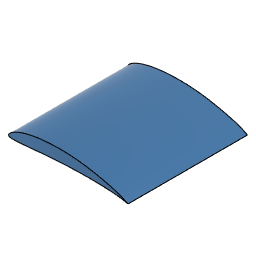
AH79100c Airfoil v1 (Autodesk Fusion 360 design; units mm, degrees)
Autodesk Fusion 360 part; units mm, degrees
sketch "AH_79-100_C_AIRFOIL_1.0" plane through (0, 0, 0) normal (0, 1, 0) x (1, 0, 0)
  spline S0 degree 5 poles (100, 0) (100.0003, -0.0014) (99.9852, -0.0078) (99.9152, -0.0286) (99.7881, -0.0733) (99.6465, -0.1452) (99.4909, -0.2271) (99.3022, -0.3153) (99.0882, -0.4084) (98.8641, -0.5062) (98.6365, -0.6097) (98.4042, -0.7199) (98.1633, -0.8374) (97.9114, -0.9618) (97.649, -1.0915) (97.3779, -1.2244) (97.1, -1.3589) (96.8164, -1.4941) (96.527, -1.6299) (96.2315, -1.7664) (95.9296, -1.9037) (95.6211, -2.0415) (95.3062, -2.1791) (94.9853, -2.3159) (94.6587, -2.4513) (94.3268, -2.5849) (93.9898, -2.7169) (93.6478, -2.8474) (93.3009, -2.9767) (92.9492, -3.1051) (92.5929, -3.2325) (92.2321, -3.359) (91.867, -3.4845) (91.4977, -3.6088) (91.1244, -3.7319) (90.7472, -3.854) (90.3662, -3.9753) (89.9815, -4.096) (89.5933, -4.2164) (89.2015, -4.3365) (88.8063, -4.4563) (88.4078, -4.5759) (88.0061, -4.6951) (87.6012, -4.8137) (87.1932, -4.9318) (86.7822, -5.0492) (86.3683, -5.166) (85.9515, -5.2822) (85.532, -5.3979) (85.1098, -5.5131) (84.6848, -5.6277) (84.2573, -5.7418) (83.8272, -5.8553) (83.3947, -5.9681) (82.9596, -6.0802) (82.5222, -6.1916) (82.0824, -6.3022) (81.6404, -6.4121) (81.1961, -6.5214) (80.7496, -6.6301) (80.3011, -6.7381) (79.8505, -6.8456) (79.3978, -6.9525) (78.9432, -7.0587) (78.4866, -7.1642) (78.0281, -7.269) (77.5676, -7.3728) (77.1054, -7.4759) (76.6413, -7.578) (76.1754, -7.6792) (75.7078, -7.7796) (75.2385, -7.8791) (74.7677, -7.9778) (74.2952, -8.0757) (73.8212, -8.1727) (73.3457, -8.2689) (72.8687, -8.3641) (72.3903, -8.4584) (71.9105, -8.5518) (71.4293, -8.6441) (70.9468, -8.7353) (70.4629, -8.8255) (69.9778, -8.9146) (69.4915, -9.0026) (69.0039, -9.0894) (68.5152, -9.175) (68.0252, -9.2594) (67.5342, -9.3427) (67.0421, -9.4247) (66.5489, -9.5056) (66.0547, -9.5851) (65.5594, -9.6634) (65.0632, -9.7403) (64.5661, -9.8157) (64.068, -9.8896) (63.5691, -9.9619) (63.0694, -10.0326) (62.5688, -10.1016) (62.0674, -10.1688) (61.5653, -10.2344) (61.0624, -10.2983) (60.5588, -10.3605) (60.0546, -10.4212) (59.5496, -10.4802) (59.0441, -10.5377) (58.5379, -10.5935) (58.0312, -10.6477) (57.5239, -10.7) (57.0162, -10.7506) (56.508, -10.7992) (55.9994, -10.8459) (55.4904, -10.8906) (54.9811, -10.9333) (54.4715, -10.9741) (53.9615, -11.0129) (53.4513, -11.0498) (52.9408, -11.0848) (52.43, -11.1179) (51.9191, -11.1491) (51.4081, -11.1784) (50.8968, -11.2059) (50.3855, -11.2314) (49.8741, -11.2551) (49.3627, -11.277) (48.8513, -11.2969) (48.3399, -11.3151) (47.8286, -11.3314) (47.3174, -11.3459) (46.8063, -11.3587) (46.2954, -11.3697) (45.7846, -11.3789) (45.2741, -11.3865) (44.7638, -11.3923) (44.2537, -11.3964) (43.7439, -11.3988) (43.2344, -11.3996) (42.7252, -11.3986) (42.2164, -11.3958) (41.7081, -11.3913) (41.2002, -11.3851) (40.6928, -11.377) (40.1859, -11.3672) (39.6797, -11.3556) (39.174, -11.3423) (38.6689, -11.3273) (38.1645, -11.3106) (37.6608, -11.2924) (37.1578, -11.2725) (36.6555, -11.251) (36.1539, -11.2279) (35.6531, -11.203) (35.1531, -11.1763) (34.6541, -11.1477) (34.1559, -11.1172) (33.6587, -11.0846) (33.1624, -11.0501) (32.6672, -11.0137) (32.173, -10.9756) (31.6799, -10.9357) (31.1879, -10.8944) (30.6971, -10.8515) (30.2074, -10.807) (29.7189, -10.7609) (29.2317, -10.7131) (28.7457, -10.6632) (28.2611, -10.6114) (27.7779, -10.5573) (27.2961, -10.501) (26.8158, -10.4427) (26.337, -10.3823) (25.8596, -10.3201) (25.3838, -10.2563) (24.9096, -10.1908) (24.4371, -10.1238) (23.9662, -10.0552) (23.497, -9.9848) (23.0297, -9.9125) (22.5643, -9.8381) (22.1008, -9.7615) (21.6392, -9.6827) (21.1797, -9.6016) (20.7223, -9.5186) (20.2669, -9.4335) (19.8136, -9.3467) (19.3624, -9.2581) (18.9135, -9.1677) (18.4668, -9.0754) (18.0225, -8.9811) (17.5806, -8.8845) (17.1412, -8.7856) (16.7044, -8.6842) (16.2702, -8.5806) (15.8386, -8.4748) (15.4097, -8.3672) (14.9835, -8.258) (14.5601, -8.1472) (14.1395, -8.0348) (13.7219, -7.9204) (13.3073, -7.8039) (12.8959, -7.6846) (12.4879, -7.5624) (12.0833, -7.4372) (11.6822, -7.309) (11.2846, -7.1782) (10.8906, -7.0453) (10.5002, -6.9106) (10.1134, -6.7744) (9.7304, -6.6366) (9.3514, -6.497) (8.9764, -6.3551) (8.6057, -6.2106) (8.2394, -6.063) (7.8776, -5.9127) (7.5203, -5.7597) (7.1675, -5.6047) (6.8194, -5.448) (6.476, -5.2898) (6.1377, -5.1298) (5.8046, -4.9676) (5.4772, -4.8025) (5.1556, -4.6344) (4.8402, -4.4631) (4.5307, -4.2897) (4.2272, -4.115) (3.9296, -3.9399) (3.6382, -3.7646) (3.3533, -3.5883) (3.076, -3.4089) (2.807, -3.2248) (2.547, -3.0352) (2.2959, -2.8413) (2.0534, -2.6463) (1.8189, -2.4534) (1.5925, -2.2645) (1.3751, -2.0779) (1.1685, -1.8892) (0.9744, -1.6949) (0.7938, -1.4952) (0.6261, -1.2977) (0.4709, -1.111) (0.329, -0.9385) (0.205, -0.769) (0.1054, -0.5848) (0.0361, -0.3768) (-0.0015, -0.1586) (-0.0069, 0.0464) (0.022, 0.2222) (0.0909, 0.3715) (0.2017, 0.5035) (0.3471, 0.6259) (0.516, 0.7423) (0.7017, 0.8506) (0.9036, 0.9444) (1.1226, 1.0187) (1.3577, 1.0749) (1.6061, 1.1191) (1.8648, 1.1579) (2.1321, 1.1941) (2.4076, 1.2263) (2.6914, 1.2522) (2.9835, 1.2698) (3.2837, 1.2798) (3.5913, 1.2839) (3.9053, 1.2845) (4.2254, 1.2832) (4.5511, 1.2802) (4.8824, 1.2754) (5.2192, 1.2681) (5.5614, 1.258) (5.9089, 1.2453) (6.2613, 1.2305) (6.6186, 1.2141) (6.9804, 1.1964) (7.3465, 1.1775) (7.7168, 1.1571) (8.0911, 1.1349) (8.4693, 1.1106) (8.8514, 1.0843) (9.2373, 1.0562) (9.6269, 1.027) (10.0201, 0.9973) (10.4168, 0.9676) (10.817, 0.938) (11.2206, 0.9083) (11.6273, 0.8778) (12.0372, 0.8459) (12.4501, 0.812) (12.8658, 0.7758) (13.2844, 0.7374) (13.7058, 0.6972) (14.1298, 0.6558) (14.5566, 0.6137) (14.9859, 0.5714) (15.4179, 0.5291) (15.8523, 0.4868) (16.2892, 0.4444) (16.7285, 0.4017) (17.1702, 0.3587) (17.6141, 0.3151) (18.0602, 0.2712) (18.5085, 0.227) (18.959, 0.1827) (19.4115, 0.1385) (19.866, 0.0945) (20.3225, 0.0507) (20.781, 0.007) (21.2414, -0.0367) (21.7036, -0.0806) (22.1677, -0.1249) (22.6335, -0.1695) (23.1011, -0.2144) (23.5703, -0.2596) (24.0412, -0.3049) (24.5137, -0.3501) (24.9878, -0.395) (25.4634, -0.4395) (25.9406, -0.4837) (26.4191, -0.5275) (26.8991, -0.5711) (27.3805, -0.6146) (27.8631, -0.658) (28.3471, -0.7014) (28.8323, -0.7447) (29.3188, -0.788) (29.8064, -0.831) (30.2952, -0.8738) (30.7852, -0.9162) (31.2763, -0.9581) (31.7685, -0.9995) (32.2617, -1.0405) (32.756, -1.081) (33.2512, -1.121) (33.7474, -1.1607) (34.2446, -1.2001) (34.7426, -1.2392) (35.2415, -1.2779) (35.7412, -1.3163) (36.2417, -1.3543) (36.743, -1.3918) (37.2449, -1.4288) (37.7476, -1.4652) (38.251, -1.501) (38.755, -1.5362) (39.2597, -1.5708) (39.765, -1.6046) (40.2709, -1.6379) (40.7774, -1.6704) (41.2844, -1.7023) (41.7919, -1.7337) (42.2999, -1.7644) (42.8083, -1.7945) (43.317, -1.8241) (43.8262, -1.8532) (44.3356, -1.8816) (44.8454, -1.9095) (45.3554, -1.9366) (45.8657, -1.9631) (46.3762, -1.9888) (46.8869, -2.0138) (47.3978, -2.038) (47.9088, -2.0616) (48.42, -2.0845) (48.9313, -2.1069) (49.4427, -2.1287) (49.9541, -2.1502) (50.4656, -2.1712) (50.977, -2.1919) (51.4883, -2.2121) (51.9996, -2.2317) (52.5108, -2.2509) (53.0219, -2.2694) (53.5328, -2.2873) (54.0435, -2.3046) (54.554, -2.3212) (55.0643, -2.3374) (55.5743, -2.353) (56.0841, -2.3682) (56.5936, -2.383) (57.1028, -2.3974) (57.6116, -2.4114) (58.12, -2.4247) (58.628, -2.4375) (59.1355, -2.4495) (59.6425, -2.4608) (60.149, -2.4713) (60.6549, -2.481) (61.1602, -2.4899) (61.665, -2.4983) (62.169, -2.506) (62.6725, -2.5134) (63.1752, -2.5203) (63.6773, -2.5268) (64.1786, -2.5328) (64.6791, -2.5383) (65.1789, -2.5432) (65.6778, -2.5474) (66.1758, -2.5508) (66.673, -2.5534) (67.1692, -2.5551) (67.6644, -2.556) (68.1586, -2.5561) (68.6518, -2.5555) (69.144, -2.5541) (69.635, -2.5521) (70.1249, -2.5495) (70.6136, -2.5462) (71.1012, -2.5423) (71.5875, -2.5378) (72.0726, -2.5326) (72.5564, -2.5268) (73.0389, -2.5202) (73.52, -2.5129) (73.9997, -2.5048) (74.478, -2.4959) (74.9548, -2.4862) (75.43, -2.4756) (75.9037, -2.4642) (76.3758, -2.4519) (76.8462, -2.4387) (77.315, -2.4248) (77.7819, -2.4101) (78.2471, -2.3946) (78.7104, -2.3784) (79.1719, -2.3613) (79.6314, -2.3435) (80.089, -2.325) (80.5445, -2.3056) (80.9981, -2.2855) (81.4495, -2.2645) (81.8989, -2.2428) (82.346, -2.2202) (82.7909, -2.1968) (83.2334, -2.1725) (83.6736, -2.1473) (84.1114, -2.1212) (84.5466, -2.094) (84.9793, -2.0658) (85.4094, -2.0365) (85.8368, -2.0063) (86.2615, -1.9751) (86.6834, -1.9431) (87.1025, -1.9104) (87.5186, -1.8772) (87.9318, -1.8433) (88.3418, -1.8088) (88.7486, -1.7734) (89.1522, -1.737) (89.5522, -1.6995) (89.9488, -1.6608) (90.3417, -1.621) (90.7311, -1.5802) (91.1167, -1.5387) (91.4985, -1.4966) (91.8765, -1.4539) (92.2504, -1.4106) (92.6201, -1.3665) (92.9854, -1.3212) (93.3461, -1.2746) (93.702, -1.2266) (94.0532, -1.1776) (94.3996, -1.1279) (94.7411, -1.0776) (95.0774, -1.0271) (95.4082, -0.976) (95.7329, -0.9239) (96.0509, -0.8705) (96.3621, -0.8157) (96.6666, -0.7597) (96.9651, -0.7034) (97.2577, -0.6475) (97.5438, -0.592) (97.8215, -0.5361) (98.0881, -0.4784) (98.342, -0.418) (98.5844, -0.355) (98.8197, -0.2919) (99.0504, -0.2315) (99.2724, -0.1758) (99.4712, -0.1252) (99.6366, -0.0793) (99.7833, -0.0381) (99.9117, -0.0107) (99.9833, 0.0007) (99.9997, 0.0014) (100, 0) knots 0 0 0 0 0 0 0.00208333 0.00416667 0.00625 0.00833333 0.01041667 0.0125 0.01458333 0.01666667 0.01875 0.02083333 0.02291667 0.025 0.02708333 0.02916667 0.03125 0.03333333 0.03541667 0.0375 0.03958333 0.04166667 0.04375 0.04583333 0.04791667 0.05 0.05208333 0.05416667 0.05625 0.05833333 0.06041667 0.0625 0.06458333 0.06666667 0.06875 0.07083333 0.07291667 0.075 0.07708333 0.07916667 0.08125 0.08333333 0.08541667 0.0875 0.08958333 0.09166667 0.09375 0.09583333 0.09791667 0.1 0.10208333 0.10416667 0.10625 0.10833333 0.11041667 0.1125 0.11458333 0.11666667 0.11875 0.12083333 0.12291667 0.125 0.12708333 0.12916667 0.13125 0.13333333 0.13541667 0.1375 0.13958333 0.14166667 0.14375 0.14583333 0.14791667 0.15 0.15208333 0.15416667 0.15625 0.15833333 0.16041667 0.1625 0.16458333 0.16666667 0.16875 0.17083333 0.17291667 0.175 0.17708333 0.17916667 0.18125 0.18333333 0.18541667 0.1875 0.18958333 0.19166667 0.19375 0.19583333 0.19791667 0.2 0.20208333 0.20416667 0.20625 0.20833333 0.21041667 0.2125 0.21458333 0.21666667 0.21875 0.22083333 0.22291667 0.225 0.22708333 0.22916667 0.23125 0.23333333 0.23541667 0.2375 0.23958333 0.24166667 0.24375 0.24583333 0.24791667 0.25 0.25208333 0.25416667 0.25625 0.25833333 0.26041667 0.2625 0.26458333 0.26666667 0.26875 0.27083333 0.27291667 0.275 0.27708333 0.27916667 0.28125 0.28333333 0.28541667 0.2875 0.28958333 0.29166667 0.29375 0.29583333 0.29791667 0.3 0.30208333 0.30416667 0.30625 0.30833333 0.31041667 0.3125 0.31458333 0.31666667 0.31875 0.32083333 0.32291667 0.325 0.32708333 0.32916667 0.33125 0.33333333 0.33541667 0.3375 0.33958333 0.34166667 0.34375 0.34583333 0.34791667 0.35 0.35208333 0.35416667 0.35625 0.35833333 0.36041667 0.3625 0.36458333 0.36666667 0.36875 0.37083333 0.37291667 0.375 0.37708333 0.37916667 0.38125 0.38333333 0.38541667 0.3875 0.38958333 0.39166667 0.39375 0.39583333 0.39791667 0.4 0.40208333 0.40416667 0.40625 0.40833333 0.41041667 0.4125 0.41458333 0.41666667 0.41875 0.42083333 0.42291667 0.425 0.42708333 0.42916667 0.43125 0.43333333 0.43541667 0.4375 0.43958333 0.44166667 0.44375 0.44583333 0.44791667 0.45 0.45208333 0.45416667 0.45625 0.45833333 0.46041667 0.4625 0.46458333 0.46666667 0.46875 0.47083333 0.47291667 0.475 0.47708333 0.47916667 0.48125 0.48333333 0.48541667 0.4875 0.48958333 0.49166667 0.49375 0.49583333 0.49791667 0.5 0.50208333 0.50416667 0.50625 0.50833333 0.51041667 0.5125 0.51458333 0.51666667 0.51875 0.52083333 0.52291667 0.525 0.52708333 0.52916667 0.53125 0.53333333 0.53541667 0.5375 0.53958333 0.54166667 0.54375 0.54583333 0.54791667 0.55 0.55208333 0.55416667 0.55625 0.55833333 0.56041667 0.5625 0.56458333 0.56666667 0.56875 0.57083333 0.57291667 0.575 0.57708333 0.57916667 0.58125 0.58333333 0.58541667 0.5875 0.58958333 0.59166667 0.59375 0.59583333 0.59791667 0.6 0.60208333 0.60416667 0.60625 0.60833333 0.61041667 0.6125 0.61458333 0.61666667 0.61875 0.62083333 0.62291667 0.625 0.62708333 0.62916667 0.63125 0.63333333 0.63541667 0.6375 0.63958333 0.64166667 0.64375 0.64583333 0.64791667 0.65 0.65208333 0.65416667 0.65625 0.65833333 0.66041667 0.6625 0.66458333 0.66666667 0.66875 0.67083333 0.67291667 0.675 0.67708333 0.67916667 0.68125 0.68333333 0.68541667 0.6875 0.68958333 0.69166667 0.69375 0.69583333 0.69791667 0.7 0.70208333 0.70416667 0.70625 0.70833333 0.71041667 0.7125 0.71458333 0.71666667 0.71875 0.72083333 0.72291667 0.725 0.72708333 0.72916667 0.73125 0.73333333 0.73541667 0.7375 0.73958333 0.74166667 0.74375 0.74583333 0.74791667 0.75 0.75208333 0.75416667 0.75625 0.75833333 0.76041667 0.7625 0.76458333 0.76666667 0.76875 0.77083333 0.77291667 0.775 0.77708333 0.77916667 0.78125 0.78333333 0.78541667 0.7875 0.78958333 0.79166667 0.79375 0.79583333 0.79791667 0.8 0.80208333 0.80416667 0.80625 0.80833333 0.81041667 0.8125 0.81458333 0.81666667 0.81875 0.82083333 0.82291667 0.825 0.82708333 0.82916667 0.83125 0.83333333 0.83541667 0.8375 0.83958333 0.84166667 0.84375 0.84583333 0.84791667 0.85 0.85208333 0.85416667 0.85625 0.85833333 0.86041667 0.8625 0.86458333 0.86666667 0.86875 0.87083333 0.87291667 0.875 0.87708333 0.87916667 0.88125 0.88333333 0.88541667 0.8875 0.88958333 0.89166667 0.89375 0.89583333 0.89791667 0.9 0.90208333 0.90416667 0.90625 0.90833333 0.91041667 0.9125 0.91458333 0.91666667 0.91875 0.92083333 0.92291667 0.925 0.92708333 0.92916667 0.93125 0.93333333 0.93541667 0.9375 0.93958333 0.94166667 0.94375 0.94583333 0.94791667 0.95 0.95208333 0.95416667 0.95625 0.95833333 0.96041667 0.9625 0.96458333 0.96666667 0.96875 0.97083333 0.97291667 0.975 0.97708333 0.97916667 0.98125 0.98333333 0.98541667 0.9875 0.98958333 0.99166667 0.99375 0.99583333 0.99791667 1 1 1 1 1 1
  point P0 (99.893, -0.038)
  point P1 (99.572, -0.184)
  point P2 (99.039, -0.43)
  point P3 (98.296, -0.773)
  point P4 (97.347, -1.239)
  point P5 (96.194, -1.783)
  point P6 (94.844, -2.374)
  point P7 (93.301, -2.976)
  point P8 (91.573, -3.583)
  point P9 (89.668, -4.193)
  point P10 (87.592, -4.816)
  point P11 (85.355, -5.446)
  point P12 (82.967, -6.078)
  point P13 (80.438, -6.705)
  point P14 (77.779, -7.325)
  point P15 (75, -7.929)
  point P16 (72.114, -8.512)
  point P17 (69.134, -9.066)
  point P18 (66.072, -9.582)
  point P19 (62.941, -10.05)
  point P20 (59.755, -10.456)
  point P21 (56.526, -10.797)
  point P22 (53.27, -11.062)
  point P23 (50, -11.249)
  point P24 (46.73, -11.36)
  point P25 (43.474, -11.399)
  point P26 (40.245, -11.368)
  point P27 (37.059, -11.268)
  point P28 (33.928, -11.102)
  point P29 (30.866, -10.866)
  point P30 (27.886, -10.569)
  point P31 (25, -10.203)
  point P32 (22.221, -9.781)
  point P33 (19.562, -9.297)
  point P34 (17.033, -8.76)
  point P35 (14.645, -8.169)
  point P36 (12.408, -7.537)
  point P37 (10.332, -6.851)
  point P38 (8.427, -6.138)
  point P39 (6.699, -5.392)
  point P40 (5.156, -4.633)
  point P41 (3.806, -3.865)
  point P42 (2.653, -3.111)
  point P43 (1.704, -2.357)
  point P44 (0.961, -1.676)
  point P45 (0.428, -1.058)
  point P46 (0.107, -0.565)
  point P47 (0.107, 0.376)
  point P48 (0.428, 0.679)
  point P49 (0.961, 0.96)
  point P50 (1.704, 1.133)
  point P51 (2.653, 1.247)
  point P52 (3.806, 1.284)
  point P53 (5.156, 1.269)
  point P54 (6.699, 1.21)
  point P55 (8.427, 1.113)
  point P56 (10.332, 0.974)
  point P57 (12.408, 0.815)
  point P58 (14.645, 0.605)
  point P59 (17.033, 0.372)
  point P60 (19.562, 0.124)
  point P61 (22.221, -0.13)
  point P62 (25, -0.396)
  point P63 (27.886, -0.66)
  point P64 (30.866, -0.923)
  point P65 (33.928, -1.175)
  point P66 (37.059, -1.415)
  point P67 (40.245, -1.636)
  point P68 (43.474, -1.833)
  point P69 (46.73, -2.006)
  point P70 (50, -2.152)
  point P71 (53.27, -2.278)
  point P72 (56.526, -2.381)
  point P73 (59.755, -2.463)
  point P74 (62.941, -2.517)
  point P75 (66.072, -2.55)
  point P76 (69.134, -2.554)
  point P77 (72.114, -2.532)
  point P78 (75, -2.485)
  point P79 (77.779, -2.41)
  point P80 (80.438, -2.31)
  point P81 (82.967, -2.187)
  point P82 (85.355, -2.04)
  point P83 (87.592, -1.871)
  point P84 (89.668, -1.688)
  point P85 (91.573, -1.488)
  point P86 (93.301, -1.28)
  point P87 (94.844, -1.062)
  point P88 (96.194, -0.845)
  point P89 (97.347, -0.63)
  point P90 (98.296, -0.428)
  point P91 (99.039, -0.235)
  point P92 (99.572, -0.097)
  point P93 (99.893, -0.016)
extrude "Extrude1" add sketch "AH_79-100_C_AIRFOIL_1.0" along normal blind 100
